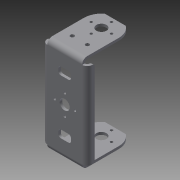
# Autodesk Inventor part: metalf5
Saved by Autodesk Inventor 2013 (Build 170138000, 138)
## iProperties
Created: 2013-09-17
Part Number: metalf5
Material: Generic
Document SubType Name: Sheet Metal
Designer: darkb_000
Density: 1 g/cm^3
Sheet Metal Rule: Default
Mass: 9.23173 g
Surface Area: 104.475 cm^2
Volume: 9.23173 cm^3
Author: darkb_000
Autodesk Inventor part; units mm, degrees
ref_plane "YZ Plane" through (0, 0, 0) normal (1, 0, 0) x (0, 1, 0)
ref_plane "XZ Plane" through (0, 0, 0) normal (0, 1, 0) x (-1, 0, 0)
ref_plane "XY Plane" through (0, 0, 0) normal (0, 0, 1) x (1, 0, 0)
sketch "Sketch1" plane through (0, 0, 0) normal (0, 0, 1) x (1, 0, 0)
  line L0 (0, -8) -> (0, -67)
  line L1 (27.5, -8) -> (27.5, -67)
  line L2 (18.75, 0) -> (27.5, 0)
  line L3 (18.75, -78) -> (27.5, -78)
  line L4 (0, -37.5) -> (0, -1.5)
  line L5 (0, -1.5) -> (27.5, -1.5)
  line L6 (27.5, -1.5) -> (27.5, -37.5)
  line L7 (0, -1.5) -> (27.5, -1.5)
  line L8 (27.5, -1.5) -> (27.5, -73.5)
  line L9 (27.5, -73.5) -> (0, -73.5)
  line L10 (0, -73.5) -> (0, -1.5)
  circle A0 centre (13.75, -37.5) radius 4
  circle A1 centre (13.75, -29.5) radius 1
  circle A2 centre (21.75, -37.5) radius 1
  circle A3 centre (5.75, -37.5) radius 1
  circle A4 centre (13.75, -45.5) radius 1
  point P0 (0, 0)
  dimension "d0" = 36
  dimension "d1" = 72
  dimension "d3" = 8
  dimension "d4" = 2
  dimension "d5" = 2
  dimension "d6" = 2
  dimension "d7" = 2
  measures "d0" distance of L4.start L4.end
  measures "d1" distance of L7.end L8.end
  measures "d3" diameter of A0
  measures "d4" diameter of A1
  measures "d5" diameter of A2
  measures "d6" diameter of A3
  measures "d7" diameter of A4
extrude "Plate1" add sketch "Sketch1" along normal blind 2
sketch "Sketch2" plane through (27.5, -1.5, 0) normal (0, 1, 0) x (-1, 0, 0)
  line L0 (27.5, 0) -> (0, 0)
  line L1 (0, 0) -> (0, -38)
  line L2 (0, -38) -> (27.5, -38)
  line L3 (27.5, -38) -> (27.5, 0)
  constraints: 6 end point, 1 horizontal, 1 perpendicular, 1 vertical
edge flange "Flange1" height 40 angle 90 thickness 2 bend radius 2 thickness toward (0, 1, 0) relief straight relief width 2 relief depth 1 edges at (13.75, -1.5, 0) wall of the first edge with corners at (0, -1.5, 0) (27.5, -1.5, 0) (27.5, -1.5, -38) (0, -1.5, -38)
bend "Bend1"
corner "Corner1"
sketch "Sketch3" plane through (0, -73.5, 0) normal (0, -1, 0) x (1, 0, 0)
  line L0 (27.5, 0) -> (0, 0)
  line L1 (0, 0) -> (0, -38)
  line L2 (0, -38) -> (27.5, -38)
  line L3 (27.5, -38) -> (27.5, 0)
  constraints: 6 end point, 1 horizontal, 1 perpendicular, 1 vertical
edge flange "Flange2" height 40 angle 90 thickness 2 bend radius 2 thickness toward (0, -1, 0) relief straight relief width 2 relief depth 1 edges at (13.75, -73.5, 0) wall of the first edge with corners at (27.5, -73.5, 0) (0, -73.5, 0) (0, -73.5, -38) (27.5, -73.5, -38)
bend "Bend2"
corner "Corner2"
sketch "Sketch4" plane through (29.5, -71.5, -2) normal (1, 0, 0) x (0, 1, 0)
  line L0 (68, 0) -> (0, 0)
  line L1 (0, 0) -> (0, -2)
  line L2 (0, -2) -> (68, -2)
  line L3 (68, -2) -> (68, 0)
  constraints: 6 end point, 1 horizontal, 1 perpendicular, 1 vertical
edge flange "Flange3" height 6 angle 90 thickness 2 bend radius 2 thickness toward (1, 0, 0) relief straight relief width 2 relief depth 1 edges at (27.5, -37.5, 0) wall of the first edge with corners at (29.5, -3.5, -2) (29.5, -71.5, -2) (29.5, -71.5, -4) (29.5, -3.5, -4)
bend "Bend3"
corner "Corner3"
sketch "Sketch5" plane through (-2, -3.5, -2) normal (-1, 0, 0) x (0, -1, 0)
  line L0 (68, 0) -> (0, 0)
  line L1 (0, 0) -> (0, -2)
  line L2 (0, -2) -> (68, -2)
  line L3 (68, -2) -> (68, 0)
  constraints: 6 end point, 1 horizontal, 1 perpendicular, 1 vertical
edge flange "Flange4" height 6 angle 90 thickness 2 bend radius 2 thickness toward (-1, 0, 0) relief straight relief width 2 relief depth 1 edges at (0, -37.5, 0) wall of the first edge with corners at (-2, -71.5, -2) (-2, -3.5, -2) (-2, -3.5, -4) (-2, -71.5, -4)
bend "Bend4"
corner "Corner4"
fillet "Corner Round1" radius 2 4 edges at (-3, -71.5, -4) (-3, -3.5, -4) (30.5, -3.5, -4) (30.5, -71.5, -4)
sketch "Sketch6" plane through (0, -75.5, -38) normal (0, -1, 0) x (1, 0, 0)
  line L0 (0, 0) -> (0, 36) projected
  line L1 (27.5, 0) -> (0, 0) projected
  line L2 (27.5, 36) -> (27.5, 0) projected
  circle A0 centre (13.75, 11) radius 13.75
  circle A1 centre (13.75, 19) radius 1
  circle A2 centre (21.75, 11) radius 1
  circle A3 centre (5.75, 11) radius 1
  circle A4 centre (13.75, 3) radius 1
  circle A5 centre (13.75, 11) radius 4
  line L3 (5.5, 0) -> (0, 0)
  line L4 (0, 11) -> (0, 0)
  line L5 (27.5, 11) -> (27.5, 0)
  line L6 (27.5, 0) -> (22, 0)
  point P0 (0, 38)
  dimension "d52" = 2
  dimension "d53" = 2
  dimension "d54" = 2
  dimension "d55" = 2
  dimension "d56" = 8
  constraints: 8 end point, 6 centre point, 4 point on circle, 4 point on line, 3 collinear, 3 tangent, 1 coincident
  measures "d52" diameter of A1
  measures "d53" diameter of A2
  measures "d54" diameter of A3
  measures "d55" diameter of A4
  measures "d56" diameter of A5
extrude "Cut1" cut sketch "Sketch6" against normal blind 2 contours L0 A0 L1 | L2 L1 A0 | A1 | A2 | A3 | A4 | A5
sketch "Sketch7" plane through (0, 0.5, -38) normal (0, 1, 0) x (1, 0, 0)
  line L0 (0, -36) -> (27.5, -36) projected
  line L1 (27.5, 0) -> (27.5, -36) projected
  line L2 (0, 0) -> (27.5, 0) projected
  line L3 (0, -36) -> (0, 0) projected
  arc A0 (27.5, -11) -> (22, 0) centre (13.75, -11) ccw projected
  line L4 (22, 0) -> (5.5, 0) projected
  arc A1 (5.5, 0) -> (0, -11) centre (13.75, -11) ccw projected
  line L5 (0, -11) -> (0, -36) projected
  line L6 (0, -36) -> (27.5, -36) projected
  line L7 (27.5, -11) -> (27.5, -36) projected
  circle A2 centre (13.75, -3) radius 1 projected
  circle A3 centre (21.75, -11) radius 1 projected
  circle A4 centre (13.75, -19) radius 1 projected
  circle A5 centre (5.75, -11) radius 1 projected
  circle A6 centre (13.75, -11) radius 4 projected
  point P0 (0, -38)
extrude "Cut2" cut sketch "Sketch7" against normal blind 2 contours L3 L2 A1 | A0 L2 L1 | A2 | A3 | A4 | A5 | A6
sketch "Sketch8" plane through (0, 0.5, -2) normal (0, 1, 0) x (1, 0, 0)
  circle A0 centre (19.75, 8) radius 1.5
  circle A1 centre (7.75, 8) radius 1.5
  point P0 (0, -2)
  dimension "d63" = 3
  dimension "d64" = 3
  constraints: 2 centre point
  measures "d63" diameter of A0
  measures "d64" diameter of A1
extrude "Cut3" cut sketch "Sketch8" against normal blind 2
sketch "Sketch9" plane through (0, -75.5, -2) normal (0, -1, 0) x (1, 0, 0)
  circle A0 centre (19.75, -8) radius 1.5 projected
  circle A1 centre (7.75, -8) radius 1.5 projected
  point P0 (0, 2)
extrude "Cut4" cut sketch "Sketch9" against normal blind 2
sketch "Sketch10" plane through (0, 0, 2) normal (0, 0, 1) x (1, 0, 0)
  circle A0 centre (13.75, -29.5) radius 1 projected
  line L0 (27.5, -3.5) -> (0, -3.5) projected
  line L1 (18.75, -59) -> (18.75, -58)
  line L2 (16.75, -56) -> (13.75, -56)
  line L3 (16.75, -56) -> (10.75, -56)
  line L4 (8.75, -58) -> (8.75, -60)
  line L5 (10.75, -62) -> (16.75, -62)
  line L6 (18.75, -60) -> (18.75, -58)
  arc A1 (8.75, -60) -> (10.75, -62) centre (10.75, -60) ccw
  arc A2 (16.75, -62) -> (18.75, -60) centre (16.75, -60) ccw
  arc A3 (10.75, -56) -> (8.75, -58) centre (10.75, -58) ccw
  arc A4 (18.75, -58) -> (16.75, -56) centre (16.75, -58) ccw
  arc A5 (18.75, -58) -> (16.75, -56) centre (16.75, -58) ccw
  line L7 (13.75, -28.5) -> (13.75, -3.5)
  line L8 (16.75, -13) -> (13.75, -13)
  line L9 (8.75, -15) -> (8.75, -17)
  line L10 (10.75, -19) -> (16.75, -19)
  line L11 (18.75, -17) -> (18.75, -15)
  arc A6 (16.75, -19) -> (18.75, -17) centre (16.75, -17) ccw
  arc A7 (8.75, -17) -> (10.75, -19) centre (10.75, -17) ccw
  arc A8 (10.75, -13) -> (8.75, -15) centre (10.75, -15) ccw
  arc A9 (18.75, -15) -> (16.75, -13) centre (16.75, -15) ccw
  line L12 (10.75, -13) -> (14.75, -13)
  point P0 (0, 0)
  point P1 (18.75, -56)
  point P2 (8.75, -62)
  point P3 (8.75, -56)
  point P4 (18.75, -62)
  point P5 (8.75, -19)
  point P6 (8.75, -13)
  dimension "d71" = 10
  dimension "d72" = 6
  dimension "d73" = 2
  dimension "d76" = 6
  dimension "d77" = 2
  constraints: 24 end point, 18 point on circle, 18 tangent, 14 point on line, 9 centre point, 7 equal radius, 3 parallel, 1 horizontal, 1 midpoint, 1 perpendicular, 1 vertical alignment, 1 other
  measures "d71" distance of point (18.75, -62) point (8.75, -62)
  measures "d72" distance of point (8.75, -62) point (8.75, -56)
  measures "d73" radius of A1
  measures "d76" distance of point (8.75, -19) point (8.75, -13)
  measures "d77" radius of A6
extrude "Cut5" cut sketch "Sketch10" against normal blind 2 contours L6 A2 L5 A1 L4 A3 L3 L2 A4 L1 | L10 A7 L9 A8 L12 L7 | L7 L8 A9 L11 A6 L10
equation "\"d57\" = Thickness"
equation "\"d59\" = Thickness"
equation "\"d65\" = Thickness"
equation "\"d67\" = Thickness"
equation "\"d78\" = Thickness"
equation "\"d9\" = BendReliefWidth"
equation "\"d10\" = BendReliefDepth"
equation "\"d11\" = MinimumRemnant"
equation "\"d12\" = BendRadius"
equation "\"d15\" = BendRadius"
equation "\"d16\" = CornerReliefSize"
equation "\"d17\" = GapSize"
equation "\"d18\" = JacobiRadiusSize"
equation "\"d19\" = BendReliefWidth"
equation "\"d20\" = BendReliefDepth"
equation "\"d21\" = MinimumRemnant"
equation "\"d22\" = BendRadius"
equation "\"d25\" = BendRadius"
equation "\"d26\" = CornerReliefSize"
equation "\"d27\" = GapSize"
equation "\"d28\" = JacobiRadiusSize"
equation "\"d29\" = BendReliefWidth"
equation "\"d30\" = BendReliefDepth"
equation "\"d31\" = MinimumRemnant"
equation "\"d32\" = BendRadius"
equation "\"d35\" = BendRadius"
equation "\"d36\" = CornerReliefSize"
equation "\"d37\" = GapSize"
equation "\"d38\" = JacobiRadiusSize"
equation "\"d39\" = BendReliefWidth"
equation "\"d40\" = BendReliefDepth"
equation "\"d41\" = MinimumRemnant"
equation "\"d42\" = BendRadius"
equation "\"d45\" = BendRadius"
equation "\"d46\" = CornerReliefSize"
equation "\"d47\" = GapSize"
equation "\"d48\" = JacobiRadiusSize"
equation "\"BendRadius\" = Thickness"
equation "\"BendReliefWidth\" = Thickness"
equation "\"BendReliefDepth\" = 0.5 * Thickness"
equation "\"CornerReliefSize\" = 4 * Thickness"
equation "\"MinimumRemnant\" = 2 * Thickness"
equation "\"TransitionRadius\" = BendRadius"
equation "\"JacobiRadiusSize\" = Thickness"
equation "\"GapSize\" = Thickness"
equation "\"d8\" = BendRadius"
equation "\"Thickness\" = 2"
body "Solid1"
